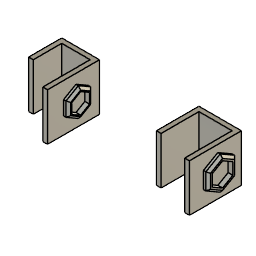
Camera Cover v1 (Autodesk Fusion 360 design; units mm, degrees)
Autodesk Fusion 360 part; units mm, degrees
sketch "Sketch1" plane through (0, 0, 0) normal (0, 0, 1) x (1, 0, 0)
  line L0 (0, 0) -> (0, 6)
  line L1 (0, 6) -> (6, 6)
  line L2 (6, 6) -> (6, -4)
  line L3 (6, -4) -> (7, -4)
  line L4 (7, -4) -> (7, 7)
  line L5 (7, 7) -> (-1, 7)
  line L6 (-1, 7) -> (-1, 0)
  line L7 (-1, 0) -> (0, 0)
  constraint coincident L0.start L7.end
  constraint vertical L0
  constraint perpendicular L0 L1
  constraint perpendicular L1 L2
  constraint perpendicular L2 L3
  constraint perpendicular L3 L4
  constraint perpendicular L4 L5
  constraint perpendicular L5 L6
  constraint perpendicular L0 L7
extrude "Extrude1" add sketch "Sketch1" along normal blind 10 makes body 1
move_body "Move1" bodies 1 to x (1, 0, 0) y (0, 1, 0) z (0, 0, 1) at (-18, 0, 0)
sketch "Sketch2" plane through (0, 0, 0) normal (0, 0, 1) x (1, 0, 0)
  line L0 (0, 0) -> (0, 8)
  line L1 (0, 8) -> (7, 8)
  line L2 (7, 8) -> (7, -2)
  line L3 (7, -2) -> (8, -2)
  line L4 (8, -2) -> (8, 9)
  line L5 (8, 9) -> (-1, 9)
  line L6 (-1, 9) -> (-1, 0)
  line L7 (-1, 0) -> (0, 0)
  constraint coincident L0.start L7.end
  constraint vertical L0
  constraint perpendicular L0 L1
  constraint perpendicular L1 L2
  constraint perpendicular L0 L3
  constraint perpendicular L3 L4
  constraint perpendicular L4 L5
  constraint perpendicular L5 L6
  constraint perpendicular L0 L7
extrude "Extrude2" add sketch "Sketch2" along normal blind 10 separate body makes body 2
sketch "Sketch3" plane through (-11, 0, 0) normal (1, 0, 0) x (0, 1, 0)
  line L0 (-4, 0) -> (7, 0)
  line L1 (7, 0) -> (7, 10)
  line L2 (7, 10) -> (-4, 10)
  line L3 (-4, 10) -> (-4, 0)
  line L4 (2, 2) -> (4.5981, 3.5)
  line L5 (4.5981, 3.5) -> (4.5981, 6.5)
  line L6 (4.5981, 6.5) -> (2, 8)
  line L7 (2, 8) -> (-0.5981, 6.5)
  line L8 (-0.5981, 6.5) -> (-0.5981, 3.5)
  line L9 (-0.5981, 3.5) -> (2, 2)
  point P0 (2, 5)
extrude "Extrude3" add sketch "Sketch3" along normal blind 1 contours L4 L5 L6 L7 L8 L9 bodies 1
sketch "Sketch4" plane through (-10, 0, 0) normal (1, 0, 0) x (0, 1, 0)
  line L0 (-0.5981, 3.5) -> (2, 2)
  line L1 (2, 2) -> (4.5981, 3.5)
  line L2 (4.5981, 3.5) -> (4.5981, 6.5)
  line L3 (4.5981, 6.5) -> (2, 8)
  line L4 (2, 8) -> (-0.5981, 6.5)
  line L5 (-0.5981, 6.5) -> (-0.5981, 3.5)
  line L6 (3.874, 6.0893) -> (1.9936, 7.1676)
  line L7 (1.9936, 7.1676) -> (0.1196, 6.0783)
  line L8 (0.1196, 6.0783) -> (0.126, 3.9107)
  line L9 (0.126, 3.9107) -> (2.0064, 2.8324)
  line L10 (2.0064, 2.8324) -> (3.8804, 3.9217)
  line L11 (3.8804, 3.9217) -> (3.874, 6.0893)
  point P0 (2, 5)
extrude "Extrude4" cut sketch "Sketch4" against normal blind 1 contours L6 L7 L8 L9 L10 L11 bodies 1
sketch "Sketch5" plane through (8, 0, 0) normal (1, 0, 0) x (0, 1, 0)
  line L0 (-2, 0) -> (9, 0)
  line L1 (9, 0) -> (9, 10)
  line L2 (9, 10) -> (-2, 10)
  line L3 (-2, 10) -> (-2, 0)
  line L4 (4, 8.5) -> (0.9689, 6.75)
  line L5 (0.9689, 6.75) -> (0.9689, 3.25)
  line L6 (0.9689, 3.25) -> (4, 1.5)
  line L7 (4, 1.5) -> (7.0311, 3.25)
  line L8 (7.0311, 3.25) -> (7.0311, 6.75)
  line L9 (7.0311, 6.75) -> (4, 8.5)
  line L10 (4, 7.5) -> (1.8349, 6.25)
  line L11 (1.8349, 6.25) -> (1.8349, 3.75)
  line L12 (1.8349, 3.75) -> (4, 2.5)
  line L13 (4, 2.5) -> (6.1651, 3.75)
  line L14 (6.1651, 3.75) -> (6.1651, 6.25)
  line L15 (6.1651, 6.25) -> (4, 7.5)
  point P0 (4, 5)
  point P1 (4, 5)
  constraint coincident P1 P0
extrude "Extrude5" add sketch "Sketch5" along normal blind 1 contours L4 L5 L6 L7 L8 L9 bodies 2
chamfer "Chamfer1" distance 0.5 angle 45 6 edges at (-10, 0.701, 7.25) (-10, -0.5981, 5) (-10, 0.701, 2.75) (-10, 3.299, 2.75) (-10, 4.5981, 5) (-10, 3.299, 7.25) on bodies 1
chamfer "Chamfer2" distance 0.5 angle 45 6 edges at (9, 2.4845, 7.625) (9, 5.5155, 7.625) (9, 0.9689, 5) (9, 2.4845, 2.375) (9, 5.5155, 2.375) (9, 7.0311, 5) on bodies 2
move_body "Move2" bodies 2 to x (1, 0, 0) y (0, 1, 0) z (0, 0, 1) at (9, 0, 0)
